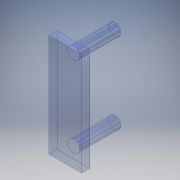
# Autodesk Inventor part: 锁销
Saved by Autodesk Inventor 2018 (Build 220112000, 112)
## iProperties
Created: 2020-11-30
Part Number: 锁销
Material: 水
Document SubType Name: Modeling
Designer: OHHHHHHHHHH
Density: 0.9983 g/cm^3
Appearance: 热带地区蓝色
Author: OHHHHHHHHHH
Autodesk Inventor part; units mm, degrees
ref_plane "YZ Plane" through (0, 0, 0) normal (1, 0, 0) x (0, 1, 0)
ref_plane "XZ Plane" through (0, 0, 0) normal (0, 1, 0) x (-1, 0, 0)
ref_plane "XY Plane" through (0, 0, 0) normal (0, 0, 1) x (1, 0, 0)
sketch "草图1" plane through (0, 0, 0) normal (0, 1, 0) x (-1, 0, 0)
  line L0 (8, 25) -> (0, 25)
  line L1 (0, 25) -> (0, 0)
  line L2 (0, 0) -> (8, 0)
  line L3 (8, 0) -> (8, 25)
  circle A0 centre (4, 22.285) radius 1.5
  line L4 (8, 12.5) -> (0, 12.5)
  line L5 (4, 25) -> (4, 0)
  circle A1 centre (4, 2.715) radius 1.5
  dimension "d0" = 25
  dimension "d1" = 8
  dimension "d2" = 3
  dimension "d6" = 19.57
  constraints: 12 end point, 4 midpoint, 2 centre point, 2 parallel, 1 horizontal, 1 perpendicular, 1 point on line, 1 symmetric about line, 1 other
  measures "d0" distance of L2.end L0.start
  measures "d1" distance of L0.start L0.end
  measures "d2" diameter of A0
  measures "d6" diameter of A0.centre L4
extrude "拉伸1" add sketch "草图1" along normal blind 10 contours L5 A0 | A0 L5 | A1 L5 | L5 A1
extrude "拉伸2" add sketch "草图1" against normal blind 2
